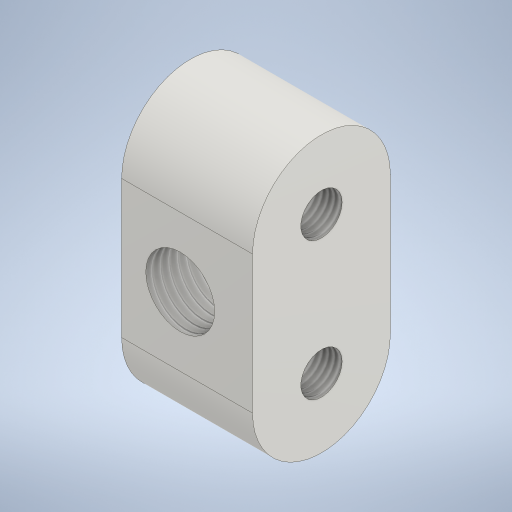
# Autodesk Inventor part: Junção Fuso
Saved by Autodesk Inventor 2024 (Build 280153000, 153)
## iProperties
Created: 2024-06-01
Part Number: Junção Fuso
Material: Steel AISI 4142 380 QT
Document SubType Name: Modeling
Designer: Pedro
Density: 7.85 g/cm^3
Appearance: Steel
Mass: 686.015 g
Surface Area: 178.262 cm^2
Volume: 87.3904 cm^3
Author: Pedro
Autodesk Inventor part; units mm, degrees
ref_plane "YZ Plane" through (0, 0, 0) normal (1, 0, 0) x (0, 1, 0)
ref_plane "XZ Plane" through (0, 0, 0) normal (0, 1, 0) x (-1, 0, 0)
ref_plane "XY Plane" through (0, 0, 0) normal (0, 0, 1) x (1, 0, 0)
sketch "Sketch2" plane through (0, 0, 0) normal (1, 0, 0) x (0, 1, 0)
  line L0 (40, 20) -> (40, -20)
  line L1 (40, -20) -> (-40, -20)
  line L2 (-40, -20) -> (-40, 20)
  line L3 (-40, 20) -> (40, 20)
  point P0 (0, 0)
  dimension "d11" = 40
  dimension "d12" = 80
  dimension "d13" = 40
  dimension "d14" = 20
  constraints: 8 end point, 2 parallel, 1 perpendicular, 1 vertical
  measures "d11" distance of L0.start L0.end
  measures "d12" distance of L0.end L1.end
  measures "d13" distance from line of point (0, 0) L0
  measures "d14" vertical distance of point (0, 0) L1.end
extrude "Extrusion2" add sketch "Sketch2" along normal blind 38
full round fillet "Full Round Fillet1" first side at (25.3333, 13.3333, 20) centre faces at (25.3333, 40, -6.6667) second side at (25.3333, -13.3333, -20)
full round fillet "Full Round Fillet2" first side at (12.6667, 0.0001, 20) centre faces at (25.3333, -40, 6.6667) second side at (12.6667, -20, -20)
sketch "Sketch3" plane through (38, 20, -20) normal (0, 0, -1) x (-1, 0, 0)
  circle A0 centre (21, -20) radius 10
  line L0 (38, -40) -> (38, 0) projected
  point P0 (38, -20)
  point P1 (38, -20)
  dimension "d15" = 20
  dimension "d16" = 17
  constraints: 1 centre point, 1 midpoint
  measures "d15" diameter of A0
  measures "d16" distance of point (38, -20) A0.centre
sketch "Sketch4" plane through (38, 0, 0) normal (1, 0, 0) x (0, 0, -1)
  circle A0 centre (0, -20) radius 6
  circle A1 centre (0, 20) radius 6
  point P0 (0, 0)
  dimension "d17" = 12
  dimension "d18" = 12
  dimension "d31" = 40
  dimension "d32" = 20
  constraints: 2 centre point
  measures "d17" diameter of A0
  measures "d18" diameter of A1
  measures "d31" distance of A0.centre A1.centre
  measures "d32" distance of point (0, 0) A0.centre
extrude "Extrusion3" cut sketch "Sketch3" against normal blind 42
extrude "Extrusion4" cut sketch "Sketch4" against normal blind 42
thread "Thread4" size "M20x2.5" class "6H" standard "ANSI Metric M Profile" full length
thread "Thread7" size "M12x1.75" class "6H" standard "ANSI Metric M Profile" length 350
thread "Thread8" size "M12x1.75" class "6H" standard "ANSI Metric M Profile" length 350
body "Solid2"
